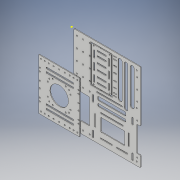
# Autodesk Inventor part: m600backplate_28Aug
Saved by Autodesk Inventor 2019 (Build 230136000, 136)
## iProperties
Created: 2019-07-14
Part Number: m600backplate_28Aug
Material: Generic
Document SubType Name: Modeling
Designer: Dell
Density: 1 g/cm^3
Appearance: Default
Author: Dell
Autodesk Inventor part; units mm, degrees
(part 1 of 2)
ref_plane "YZ Plane" through (0, 0, 0) normal (1, 0, 0) x (0, 1, 0)
ref_plane "XZ Plane" through (0, 0, 0) normal (0, 1, 0) x (-1, 0, 0)
ref_plane "XY Plane" through (0, 0, 0) normal (0, 0, 1) x (1, 0, 0)
sketch "Sketch1" plane through (0, 0, 0) normal (0, 0, 1) x (1, 0, 0)
  point P0 (0, 0)
sketch "Sketch2" plane through (0, 0, 0) normal (0, 0, 1) x (1, 0, 0)
  point P0 (0, 0)
sketch "Sketch3" plane through (0, 0, 0) normal (0, 0, 1) x (1, 0, 0)
  line L0 (0, 0) -> (190, 0)
  line L1 (190, 0) -> (190, -240)
  line L2 (190, -240) -> (0, -240)
  line L3 (0, -240) -> (0, 0)
  dimension "d0" = 190
  dimension "d1" = 240
  constraints: 8 end point, 2 parallel, 1 horizontal, 1 perpendicular
  measures "d0" distance of L1.end L2.end
  measures "d1" distance of L0.end L1.end
extrude "Extrusion1" add sketch "Sketch3" along normal blind 2
sketch "Sketch4" plane through (0, 0, 2) normal (0, 0, 1) x (1, 0, 0)
  line L0 (190, 0) -> (0, 0) projected
  line L1 (190, 0) -> (179.65, 0)
  line L2 (179.65, 0) -> (179.65, -13)
  line L3 (179.65, -13) -> (190, -13)
  line L4 (190, -13) -> (190, 0)
  line L5 (0, -240) -> (190, -240) projected
  line L6 (190, -240) -> (179.65, -240)
  line L7 (179.65, -240) -> (179.65, -230)
  line L8 (179.65, -230) -> (190, -230)
  line L9 (190, -230) -> (190, -240)
  circle A0 centre (179.65, -13) radius 1.75
  circle A1 centre (179.65, -230) radius 1.75
  line L10 (190, 0) -> (50.325, 0)
  line L11 (50.325, 0) -> (50.325, -10)
  line L12 (190, -10) -> (190, 0)
  line L13 (50.325, 0) -> (32.255, 0)
  line L14 (32.255, 0) -> (32.255, -10)
  line L15 (50.325, -10) -> (50.325, 0)
  line L16 (190, -240) -> (50.325, -240)
  line L17 (50.325, -240) -> (50.325, -230)
  line L18 (50.325, -230) -> (190, -230)
  line L19 (190, -230) -> (190, -240)
  line L20 (50.325, -240) -> (32.255, -240)
  line L21 (32.255, -240) -> (32.255, -230)
  line L22 (32.255, -230) -> (50.325, -230)
  line L23 (50.325, -230) -> (50.325, -240)
  circle A2 centre (50.325, -230) radius 1.75
  circle A3 centre (32.255, -230) radius 1.75
  line L24 (190, 0) -> (50.325, 0)
  line L25 (50.325, 0) -> (50.325, -13)
  line L26 (50.325, -13) -> (190, -13)
  line L27 (190, -13) -> (190, 0)
  line L28 (190, 0) -> (32.255, 0)
  line L29 (32.255, 0) -> (32.255, -13)
  line L30 (32.255, -13) -> (190, -13)
  line L31 (190, -13) -> (190, 0)
  circle A4 centre (32.255, -13) radius 1.75
  circle A5 centre (50.325, -13) radius 1.75
  line L32 (32.255, -13) -> (15.255, -13)
  circle A6 centre (15.255, -13) radius 1.75
  line L33 (190, -13) -> (179.65, -13)
  line L34 (179.65, -13) -> (179.65, -43)
  line L35 (179.65, -43) -> (190, -43)
  line L36 (190, -43) -> (190, -13)
  line L37 (179.65, -13) -> (50.325, -13)
  line L38 (50.325, -13) -> (50.325, -42.7133)
  line L39 (50.325, -42.7133) -> (179.65, -42.7133)
  line L40 (179.65, -42.7133) -> (179.65, -13)
  line L41 (50.325, -13) -> (32.255, -13)
  line L42 (32.255, -13) -> (32.255, -42.7133)
  line L43 (32.255, -42.7133) -> (50.325, -42.7133)
  line L44 (50.325, -42.7133) -> (50.325, -13)
  line L45 (32.255, -13) -> (15.255, -13)
  line L46 (15.255, -13) -> (15.255, -42.7133)
  line L47 (15.255, -42.7133) -> (32.255, -42.7133)
  line L48 (32.255, -42.7133) -> (32.255, -13)
  line L49 (190, -43) -> (179.65, -43)
  line L50 (179.65, -43) -> (179.65, -73)
  line L51 (179.65, -73) -> (190, -73)
  line L52 (190, -73) -> (190, -43)
  line L53 (179.65, -43) -> (50.325, -43)
  line L54 (50.325, -43) -> (50.325, -73)
  line L55 (50.325, -73) -> (179.65, -73)
  line L56 (179.65, -73) -> (179.65, -43)
  line L57 (50.325, -43) -> (32.255, -43)
  line L58 (32.255, -43) -> (32.255, -73)
  line L59 (32.255, -73) -> (50.325, -73)
  line L60 (50.325, -73) -> (50.325, -43)
  line L61 (32.255, -43) -> (15.255, -43)
  line L62 (15.255, -43) -> (15.255, -73)
  line L63 (15.255, -73) -> (32.255, -73)
  line L64 (32.255, -73) -> (32.255, -43)
  line L65 (190, -73) -> (179.65, -73)
  line L66 (179.65, -73) -> (179.65, -103)
  line L67 (179.65, -103) -> (190, -103)
  line L68 (190, -103) -> (190, -73)
  line L69 (179.65, -73) -> (50.325, -73)
  line L70 (50.325, -73) -> (50.325, -103)
  line L71 (50.325, -103) -> (179.65, -103)
  line L72 (179.65, -103) -> (179.65, -73)
  line L73 (50.325, -73) -> (32.255, -73)
  line L74 (32.255, -73) -> (32.255, -103)
  line L75 (32.255, -103) -> (50.325, -103)
  line L76 (50.325, -103) -> (50.325, -73)
  line L77 (32.255, -73) -> (15.255, -73)
  line L78 (15.255, -73) -> (15.255, -103)
  line L79 (15.255, -103) -> (32.255, -103)
  line L80 (32.255, -103) -> (32.255, -73)
  circle A7 centre (179.65, -43) radius 1.75
  circle A8 centre (179.65, -73) radius 1.75
  circle A9 centre (179.65, -103) radius 1.75
  circle A10 centre (50.325, -43) radius 1.75
  circle A11 centre (32.255, -43) radius 1.75
  circle A12 centre (15.255, -43) radius 1.75
  circle A13 centre (50.325, -73) radius 1.75
  circle A14 centre (32.255, -73) radius 1.75
  circle A15 centre (15.255, -73) radius 1.75
  circle A16 centre (15.255, -103) radius 1.75
  circle A17 centre (32.255, -103) radius 1.75
  circle A18 centre (50.325, -103) radius 1.75
  line L81 (50.325, -13) -> (53.325, -13)
  line L82 (53.325, -13) -> (53.325, -8)
  line L83 (53.325, -8) -> (50.325, -8)
  line L84 (50.325, -8) -> (50.325, -13)
  line L85 (53.325, -8) -> (112.325, -8)
  line L86 (112.325, -8) -> (112.325, -92.2031)
  line L87 (112.325, -92.2031) -> (53.325, -92.2031)
  line L88 (53.325, -92.2031) -> (53.325, -8)
  line L89 (53.325, -8) -> (112.325, -8)
  line L90 (112.325, -8) -> (112.325, -111)
  line L91 (112.325, -111) -> (53.325, -111)
  line L92 (53.325, -111) -> (53.325, -8)
  line L93 (50.325, -13) -> (127.325, -13)
  line L94 (127.325, -13) -> (127.325, -58)
  line L95 (127.325, -58) -> (50.325, -58)
  line L96 (50.325, -58) -> (50.325, -13)
  line L97 (127.325, -58) -> (112.325, -58)
  line L98 (112.325, -58) -> (112.325, -18.0003)
  line L99 (112.325, -18.0003) -> (127.325, -18.0003)
  line L100 (127.325, -18.0003) -> (127.325, -58)
  line L101 (127.325, -58) -> (112.325, -58)
  line L102 (112.325, -58) -> (112.325, -97.9958)
  line L103 (112.325, -97.9958) -> (127.325, -97.9958)
  line L104 (127.325, -97.9958) -> (127.325, -58)
  line L105 (116.2641, -18.0003) -> (123.5774, -18.0003) construction
  line L106 (116.2641, -19.0003) -> (123.5774, -19.0003)
  line L107 (123.5774, -17.0003) -> (116.2641, -17.0003)
  arc A19 (116.2641, -17.0003) -> (116.2641, -19.0003) centre (116.2641, -18.0003) ccw
  arc A20 (123.5774, -19.0003) -> (123.5774, -17.0003) centre (123.5774, -18.0003) ccw
  line L108 (116.2641, -97.9958) -> (123.5774, -97.9958) construction
  line L109 (116.2641, -98.9958) -> (123.5774, -98.9958)
  line L110 (123.5774, -96.9958) -> (116.2641, -96.9958)
  arc A21 (116.2641, -96.9958) -> (116.2641, -98.9958) centre (116.2641, -97.9958) ccw
  arc A22 (123.5774, -98.9958) -> (123.5774, -96.9958) centre (123.5774, -97.9958) ccw
  line L111 (116.2641, -10.5) -> (123.5774, -10.5) construction
  line L112 (116.2641, -11.5) -> (123.5774, -11.5)
  line L113 (123.5774, -9.5) -> (116.2641, -9.5)
  arc A23 (116.2641, -9.5) -> (116.2641, -11.5) centre (116.2641, -10.5) ccw
  arc A24 (123.5774, -11.5) -> (123.5774, -9.5) centre (123.5774, -10.5) ccw
  line L114 (116.2641, -104.75) -> (123.5774, -104.75) construction
  line L115 (116.2641, -105.75) -> (123.5774, -105.75)
  line L116 (123.5774, -103.75) -> (116.2641, -103.75)
  arc A25 (116.2641, -103.75) -> (116.2641, -105.75) centre (116.2641, -104.75) ccw
  arc A26 (123.5774, -105.75) -> (123.5774, -103.75) centre (123.5774, -104.75) ccw
  line L117 (50.325, -103) -> (32.255, -103)
  line L118 (32.255, -103) -> (32.255, -128)
  line L119 (32.255, -128) -> (50.325, -128)
  line L120 (50.325, -128) -> (50.325, -103)
  circle A27 centre (50.325, -128) radius 1.75
  circle A28 centre (32.255, -128) radius 1.75
  line L121 (190, -240) -> (190, 0) projected
  line L122 (190, -240) -> (181, -240)
  line L123 (181, -240) -> (181, -219.8278)
  line L124 (181, -219.8278) -> (190, -219.8278)
  line L125 (190, -219.8278) -> (190, -240)
  circle A29 centre (181, -219.8278) radius 1.75
  line L126 (116.9207, -32.9136) -> (122.9207, -32.9136) construction
  line L127 (116.9207, -34.2126) -> (122.9207, -34.2126)
  line L128 (122.9207, -31.6146) -> (116.9207, -31.6146)
  arc A30 (116.9207, -31.6146) -> (116.9207, -34.2126) centre (116.9207, -32.9136) ccw
  arc A31 (122.9207, -34.2126) -> (122.9207, -31.6146) centre (122.9207, -32.9136) ccw
  line L129 (116.9207, -49.8149) -> (122.9207, -49.8149) construction
  line L130 (116.9207, -51.1246) -> (122.9207, -51.1246)
  line L131 (122.9207, -48.5051) -> (116.9207, -48.5051)
  arc A32 (116.9207, -48.5051) -> (116.9207, -51.1246) centre (116.9207, -49.8149) ccw
  arc A33 (122.9207, -51.1246) -> (122.9207, -48.5051) centre (122.9207, -49.8149) ccw
  line L132 (116.9207, -68.5514) -> (122.9207, -68.5514) construction
  line L133 (116.9207, -69.571) -> (122.9207, -69.571)
  line L134 (122.9207, -67.5318) -> (116.9207, -67.5318)
  arc A34 (116.9207, -67.5318) -> (116.9207, -69.571) centre (116.9207, -68.5514) ccw
  arc A35 (122.9207, -69.571) -> (122.9207, -67.5318) centre (122.9207, -68.5514) ccw
  line L135 (116.9207, -84.977) -> (122.9207, -84.977) construction
  line L136 (116.9207, -86.0208) -> (122.9207, -86.0208)
  line L137 (122.9207, -83.9332) -> (116.9207, -83.9332)
  arc A36 (116.9207, -83.9332) -> (116.9207, -86.0208) centre (116.9207, -84.977) ccw
  arc A37 (122.9207, -86.0208) -> (122.9207, -83.9332) centre (122.9207, -84.977) ccw
  point P0 (119.9207, -18.0003)
  point P1 (119.9207, -97.9958)
  point P2 (119.9207, -10.5)
  point P3 (119.9207, -104.75)
  point P4 (119.9207, -32.9136)
  point P5 (119.9207, -49.8149)
  point P6 (119.9207, -68.5514)
  point P7 (119.9207, -84.977)
  dimension "d4" = 10.35
  dimension "d5" = 13
  dimension "d6" = 10.35
  dimension "d7" = 10
  dimension "d8" = 3.5
  dimension "d9" = 3.5
  dimension "d17" = 139.675
  dimension "d18" = 18.07
  dimension "d21" = 3.5
  dimension "d22" = 3.5
  dimension "d28" = 3.5
  dimension "d29" = 3.5
  dimension "d30" = 17
  dimension "d31" = 3.5
  dimension "d32" = 30
  dimension "d33" = 30
  dimension "d34" = 30
  dimension "d35" = 3.5
  dimension "d36" = 3.5
  dimension "d37" = 3.5
  dimension "d38" = 3.5
  dimension "d39" = 3.5
  dimension "d40" = 3.5
  dimension "d41" = 3.5
  dimension "d42" = 3.5
  dimension "d43" = 3.5
  dimension "d44" = 3.5
  dimension "d45" = 3.5
  dimension "d46" = 3.5
  dimension "d49" = 3
  dimension "d50" = 5
  dimension "d51" = 59
  dimension "d52" = 84.2031
  dimension "d54" = 77
  dimension "d55" = 45
  dimension "d56" = 2
  dimension "d57" = 2
  dimension "d58" = 2
  dimension "d59" = 2
  dimension "d89" = 103
  dimension "d105" = 3.5
  dimension "d106" = 3.5
  dimension "d107" = 25
  dimension "d111" = 3.5
  dimension "d112" = 9
  dimension "d148" = 6
  dimension "d149" = 6
  dimension "d150" = 7.1016
  dimension "d151" = 6
  dimension "d152" = 6
  constraints: 286 end point, 67 parallel, 38 centre point, 32 point on circle, 32 tangent, 29 horizontal, 29 perpendicular, 22 coincident, 14 point on line, 8 midpoint, 1 other
  measures "d4" distance of L3.end L2.end
  measures "d5" distance of L1.end L2.end
  measures "d6" distance of L7.end L8.end
  measures "d7" distance of L6.end L7.end
  measures "d8" diameter of A0
  measures "d9" diameter of A1
  measures "d17" distance of L12.start L11.end
  measures "d18" distance of L15.start L14.end
  measures "d21" diameter of A2
  measures "d22" diameter of A3
  measures "d28" diameter of A4
  measures "d29" diameter of A5
  measures "d30" distance of L32.start L32.end
  measures "d31" diameter of A6
  measures "d32" distance of L33.end L34.end
  measures "d33" distance of L49.end L50.end
  measures "d34" distance of L65.end L66.end
  measures "d35" diameter of A7
  measures "d36" diameter of A8
  measures "d37" diameter of A9
  measures "d38" diameter of A10
  measures "d39" diameter of A11
  measures "d40" diameter of A12
  measures "d41" diameter of A13
  measures "d42" diameter of A14
  measures "d43" diameter of A15
  measures "d44" diameter of A16
  measures "d45" diameter of A17
  measures "d46" diameter of A18
  measures "d49" distance of L83.end L82.end
  measures "d50" distance of L81.end L82.end
  measures "d51" distance of L86.end L87.end
  measures "d52" distance of L85.end L86.end
  measures "d54" distance of L94.end L95.end
  measures "d55" distance of L93.end L94.end
  measures "d56" diameter of A20
  measures "d57" diameter of A22
  measures "d58" diameter of A24
  measures "d59" diameter of A26
  measures "d89" distance of L89.end L90.end
  measures "d105" diameter of A27
  measures "d106" diameter of A28
  measures "d107" distance of L119.end L117.start
  measures "d111" diameter of A29
  measures "d112" distance of L123.end L124.end
  measures "d148" distance of L135.start L135.end
  measures "d149" distance of L132.start L132.end
  measures "d150" distance between parallel lines of L39 L129
  measures "d151" distance of L131.start L131.end
  measures "d152" distance of L126.start L126.end
extrude "Extrusion2" cut sketch "Sketch4" against normal blind 2 contours A0 L3 L2 | L2 L26 A0 | L34 A0 L26 | L3 A0 L34 | L85 L86 L26 L82 | A4 L30 L29 | L29 L32 A4 | A5 L26 L25 | L25 L30 A5 | L26 L86 L39 L88 | L42 A4 L32 | L30 A4 L42 | L38 A5 L30 | L26 A5 L38 | L39 L86 L53 L88 | A20 L106 A19 L99 | L99 A19 L107 A20 | A9 L71 L67 | L67 L66 A9 | A6 L46 L32 | L32 L46 A6 | A10 L53 L96 L39 | L39 L38 A10 | L53 L86 L95 L88 | L66 L71 A9 | A29 L123 L124 | L124 L123 A29 | A11 L43 L42 | L42 L47 A11 | L38 L43 A10 | L96 L57 A10 L43 | A10 L54 L53 | L95 L86 L55 L88 | L90 L91 L92 L71 | L71 L92 L87 L90 | A1 L123 L8 | L8 L123 A1 | L43 A11 L57 L61 L47 | A12 L47 L46 | L46 L47 A12 L61 L62 | L54 A10 L57 | L55 L86 L87 L88 | L123 A1 L7 L8 | L8 L18 A1 L123 | A11 L58 L57 | L61 L58 A11 | L62 L61 A12 | A13 L70 L55 | L55 L54 A13 | L54 L59 A13 | A22 L109 A21 L103 | L103 A21 L110 A22 | A18 L120 L71 | L71 L70 A18 | L7 A1 L18 | A15 L63 L62 | L62 L78 A15 | L70 A13 L59 | L75 A18 L70 | L120 A18 L75 | A2 L17 L18 | L18 L22 A2 | A14 L59 L58 | L58 L63 A14 | L63 A15 L78 | A14 L74 L59 | A27 L119 L120 | L120 L119 A27 | L17 A2 L22 | L74 A14 L63 | A16 L79 L78 | L78 L79 A16 | A17 L118 L75 | L75 L74 A17 | A3 L21 L22 | L22 L21 A3 | L74 L79 A17 | L118 A17 L79 | A28 L118 L119 | L119 L118 A28 | A23 L113 A24 L112 | A25 L116 A26 L115 | A30 L128 A31 L127 | A32 L131 A33 L130 | A34 L134 A35 L133 | A36 L137 A37 L136
sketch "Sketch5" plane through (0, 0, 2) normal (0, 0, 1) x (1, 0, 0)
  line L0 (190, 0) -> (190, -240) projected
  line L1 (190, 0) -> (181, 0)
  line L2 (181, 0) -> (181, -86.7053)
  line L3 (181, -86.7053) -> (190, -86.7053)
  line L4 (190, -86.7053) -> (190, 0)
  line L5 (190, -240) -> (181, -240)
  line L6 (181, -240) -> (181, -131.882)
  line L7 (181, -131.882) -> (190, -131.882)
  line L8 (190, -131.882) -> (190, -240)
  circle A0 centre (181, -86.7053) radius 1.75
  circle A1 centre (181, -131.882) radius 1.75
  line L9 (190, 0) -> (181, 0)
  line L10 (181, 0) -> (181, -28.9003)
  line L11 (181, -28.9003) -> (190, -28.9003)
  line L12 (190, -28.9003) -> (190, 0)
  line L13 (190, -28.9003) -> (181, -28.9003)
  line L14 (181, -28.9003) -> (181, -58.2669)
  line L15 (181, -58.2669) -> (190, -58.2669)
  line L16 (190, -58.2669) -> (190, -28.9003)
  circle A2 centre (181, -28.9003) radius 1.75
  circle A3 centre (181, -58.2669) radius 1.75
  point P0 (0, 0)
  dimension "d12" = 9
  dimension "d13" = 3.5
  dimension "d14" = 3.5
  dimension "d47" = 3.5
  dimension "d48" = 3.5
  constraints: 32 end point, 8 parallel, 4 centre point, 4 coincident, 4 horizontal, 4 perpendicular, 3 point on line
  measures "d12" distance of L3.end L2.end
  measures "d13" diameter of A0
  measures "d14" diameter of A1
  measures "d47" diameter of A2
  measures "d48" diameter of A3
extrude "Extrusion3" cut sketch "Sketch5" against normal blind 2 contours A2 L2 L11 | L11 L2 A2 | L2 A2 | A3 L2 L15 | L15 L2 A3 | A0 L2 L3 | L3 L2 A0 | L2 A3 | A1 L6 L7 | L7 L6 A1
sketch "Sketch6" plane through (0, 0, 2) normal (0, 0, 1) x (1, 0, 0)
  line L0 (0, 0) -> (25, 0)
  line L1 (25, 0) -> (25, -108)
  line L2 (25, -108) -> (0, -108)
  line L3 (0, -108) -> (0, 0)
  circle A0 centre (32.255, -10) radius 1.75 projected
  line L4 (0, -108) -> (25, -108)
  line L5 (25, -108) -> (25, -240)
  line L6 (25, -240) -> (0, -240)
  line L7 (0, -240) -> (0, -108)
  line L8 (190, 0) -> (0, 0) projected
  line L9 (0, 0) -> (7.255, 0)
  line L10 (7.255, 0) -> (7.255, -108)
  line L11 (7.255, -108) -> (0, -108)
  line L12 (0, -108) -> (0, 0)
  line L13 (0, 0) -> (0, -240) projected
  line L14 (0, 0) -> (50.325, 0)
  line L15 (50.325, 0) -> (50.325, -160)
  line L16 (50.325, -160) -> (0, -160)
  line L17 (0, -160) -> (0, 0)
  line L18 (0, -160) -> (50.325, -160)
  line L19 (50.325, -160) -> (50.325, -210)
  line L20 (50.325, -210) -> (0, -210)
  line L21 (0, -210) -> (0, -160)
  line L22 (190, -159.8282) -> (179.65, -159.8282)
  line L23 (179.65, -159.8282) -> (179.65, -210.3723)
  line L24 (179.65, -210.3723) -> (190, -210.3723)
  line L25 (190, -210.3723) -> (190, -159.8282)
  dimension "d23" = 108
  dimension "d24" = 25
  dimension "d53" = 7.255
  dimension "d60" = 160
  dimension "d61" = 50
  constraints: 48 end point, 12 parallel, 6 horizontal, 6 perpendicular, 1 point on line
  measures "d23" distance of L0.end L1.end
  measures "d24" distance of L1.end L2.end
  measures "d53" distance of L10.end L11.end
  measures "d60" distance of L14.end L15.end
  measures "d61" distance of L18.end L19.end
extrude "Extrusion4" cut sketch "Sketch6" against normal blind 10 contours L0 L10 L2 L3 | L2 L5 L16 L7 | L16 L5 L20 L7 | L20 L5 L6 L7 | L16 L19 L20 L5 | L25 L24 L23 L22
sketch "Sketch7" plane through (38.9808, -119.1264, 2) normal (0, 0, 1) x (1, 0, 0)
  line L0 (150, -215) -> (150, 0)
  line L1 (150, 0) -> (129.155, 0)
  line L2 (129.155, 0) -> (129.155, -12.875)
  line L3 (129.155, -12.875) -> (150, -12.875)
  line L4 (150, -12.875) -> (150, 0)
  line L5 (0, 0) -> (20.845, 0)
  line L6 (20.845, 0) -> (20.845, -12.875)
  line L7 (20.845, -12.875) -> (0, -12.875)
  line L8 (0, -12.875) -> (0, 0)
  circle A0 centre (129.155, -12.875) radius 1.75
  circle A1 centre (20.845, -12.875) radius 1.75
  line L9 (150, 0) -> (129.155, 0)
  line L10 (129.155, 0) -> (129.155, -97.755)
  line L11 (129.155, -97.755) -> (150, -97.755)
  line L12 (150, -97.755) -> (150, 0)
  line L13 (0, 0) -> (20.845, 0)
  line L14 (20.845, 0) -> (20.845, -97.755)
  line L15 (20.845, -97.755) -> (0, -97.755)
  line L16 (0, -97.755) -> (0, 0)
  circle A2 centre (20.845, -97.755) radius 1.75
  circle A3 centre (129.155, -97.755) radius 1.75
  line L17 (150, 0) -> (0, 0)
  line L18 (0, 0) -> (20.845, 0)
  line L19 (20.845, 0) -> (20.845, -27.95)
  line L20 (20.845, -27.95) -> (0, -27.95)
  line L21 (0, -27.95) -> (0, 0)
  circle A4 centre (20.845, -27.95) radius 1.75
  line L22 (150, 0) -> (129.155, 0)
  line L23 (129.155, 0) -> (129.155, -27.95)
  line L24 (129.155, -27.95) -> (150, -27.95)
  line L25 (150, -27.95) -> (150, 0)
  circle A5 centre (129.155, -27.95) radius 1.75
  line L26 (0, -97.755) -> (20.845, -97.755)
  line L27 (20.845, -97.755) -> (20.845, -112.83)
  line L28 (20.845, -112.83) -> (0, -112.83)
  line L29 (0, -112.83) -> (0, -97.755)
  line L30 (150, -97.755) -> (129.155, -97.755)
  line L31 (129.155, -97.755) -> (129.155, -112.83)
  line L32 (129.155, -112.83) -> (150, -112.83)
  line L33 (150, -112.83) -> (150, -97.755)
  circle A6 centre (20.845, -112.83) radius 1.75
  circle A7 centre (129.155, -112.83) radius 1.75
  line L34 (20.845, -12.875) -> (20.845, -27.95) construction
  line L35 (19.095, -12.875) -> (19.095, -27.95)
  line L36 (22.595, -27.95) -> (22.595, -12.875)
  arc A8 (22.595, -12.875) -> (19.095, -12.875) centre (20.845, -12.875) ccw
  arc A9 (19.095, -27.95) -> (22.595, -27.95) centre (20.845, -27.95) ccw
  line L37 (129.155, -27.95) -> (129.1553, -12.8747) construction
  line L38 (130.905, -27.95) -> (130.9053, -12.8747)
  line L39 (127.4053, -12.8746) -> (127.405, -27.95)
  arc A10 (127.405, -27.95) -> (130.905, -27.95) centre (129.155, -27.95) ccw
  arc A11 (130.9053, -12.8747) -> (127.4053, -12.8746) centre (129.1553, -12.8747) ccw
  line L40 (129.155, -97.755) -> (129.155, -112.83) construction
  line L41 (127.405, -97.755) -> (127.405, -112.83)
  line L42 (130.905, -112.83) -> (130.905, -97.755)
  arc A12 (130.905, -97.755) -> (127.405, -97.755) centre (129.155, -97.755) ccw
  arc A13 (127.405, -112.83) -> (130.905, -112.83) centre (129.155, -112.83) ccw
  line L43 (20.845, -97.755) -> (20.845, -112.83) construction
  line L44 (19.095, -97.755) -> (19.095, -112.83)
  line L45 (22.595, -112.83) -> (22.595, -97.755)
  arc A14 (22.595, -97.755) -> (19.095, -97.755) centre (20.845, -97.755) ccw
  arc A15 (19.095, -112.83) -> (22.595, -112.83) centre (20.845, -112.83) ccw
  line L46 (42.3212, -18.1679) -> (102.3212, -18.1679) construction
  line L47 (42.3212, -19.6679) -> (102.3212, -19.6679)
  line L48 (102.3212, -16.6679) -> (42.3212, -16.6679)
  arc A16 (42.3212, -16.6679) -> (42.3212, -19.6679) centre (42.3212, -18.1679) ccw
  arc A17 (102.3212, -19.6679) -> (102.3212, -16.6679) centre (102.3212, -18.1679) ccw
  arc A18 (118.7811, -14.3736) -> (118.7811, -11.3736) centre (118.7811, -12.8736) ccw
  line L49 (31.9307, 0) -> (99.9307, 0) construction
  line L50 (31.9307, -1.5) -> (99.9307, -1.5)
  line L51 (99.9307, 1.5) -> (31.9307, 1.5)
  arc A19 (31.9307, 1.5) -> (31.9307, -1.5) centre (31.9307, 0) ccw
  arc A20 (99.9307, -1.5) -> (99.9307, 1.5) centre (99.9307, 0) ccw
  line L52 (42.3212, -44.7177) -> (102.3212, -44.7177) construction
  line L53 (42.3212, -46.2177) -> (102.3212, -46.2177)
  line L54 (102.3212, -43.2177) -> (42.3212, -43.2177)
  arc A21 (42.3212, -43.2177) -> (42.3212, -46.2177) centre (42.3212, -44.7177) ccw
  arc A22 (102.3212, -46.2177) -> (102.3212, -43.2177) centre (102.3212, -44.7177) ccw
  line L55 (90.1611, 94.0299) -> (90.1611, 77.0497) construction
  line L56 (87.6611, 94.0299) -> (87.6611, 77.0497)
  line L57 (92.6611, 77.0497) -> (92.6611, 94.0299)
  arc A23 (92.6611, 94.0299) -> (87.6611, 94.0299) centre (90.1611, 94.0299) ccw
  arc A24 (87.6611, 77.0497) -> (92.6611, 77.0497) centre (90.1611, 77.0497) ccw
  line L58 (90.1611, 48.3141) -> (90.1611, 31.2392) construction
  line L59 (88.8111, 48.3141) -> (88.8111, 31.2392)
  line L60 (91.5111, 31.2392) -> (91.5111, 48.3141)
  arc A25 (91.5111, 48.3141) -> (88.8111, 48.3141) centre (90.1611, 48.3141) ccw
  arc A26 (88.8111, 31.2392) -> (91.5111, 31.2392) centre (90.1611, 31.2392) ccw
  line L61 (131.941, 94.0299) -> (131.941, 77.0497) construction
  line L62 (130.591, 94.0299) -> (130.591, 77.0497)
  line L63 (133.291, 77.0497) -> (133.291, 94.0299)
  arc A27 (133.291, 94.0299) -> (130.591, 94.0299) centre (131.941, 94.0299) ccw
  arc A28 (130.591, 77.0497) -> (133.291, 77.0497) centre (131.941, 77.0497) ccw
  line L64 (131.941, 48.3141) -> (131.941, 31.2392) construction
  line L65 (130.591, 48.3141) -> (130.591, 31.2392)
  line L66 (133.291, 31.2392) -> (133.291, 48.3141)
  arc A29 (133.291, 48.3141) -> (130.591, 48.3141) centre (131.941, 48.3141) ccw
  arc A30 (130.591, 31.2392) -> (133.291, 31.2392) centre (131.941, 31.2392) ccw
  line L67 (112.7117, 142.4796) -> (112.7117, 43.0119) construction
  line L68 (26.4237, -54.8428) -> (26.4237, -84.9666) construction
  line L69 (25.0737, -54.8428) -> (25.0737, -84.9666)
  line L70 (27.7737, -84.9666) -> (27.7737, -54.8428)
  arc A31 (27.7737, -54.8428) -> (25.0737, -54.8428) centre (26.4237, -54.8428) ccw
  arc A32 (25.0737, -84.9666) -> (27.7737, -84.9666) centre (26.4237, -84.9666) ccw
  line L71 (51.0407, -54.8428) -> (51.0407, -84.9666) construction
  line L72 (49.6907, -54.8428) -> (49.6907, -84.9666)
  line L73 (52.3907, -84.9666) -> (52.3907, -54.8428)
  arc A33 (52.3907, -54.8428) -> (49.6907, -54.8428) centre (51.0407, -54.8428) ccw
  arc A34 (49.6907, -84.9666) -> (52.3907, -84.9666) centre (51.0407, -84.9666) ccw
  line L74 (73.6712, -54.8428) -> (73.6712, -84.9666) construction
  line L75 (72.3212, -54.8428) -> (72.3212, -84.9666)
  line L76 (75.0212, -84.9666) -> (75.0212, -54.8428)
  arc A35 (75.0212, -54.8428) -> (72.3212, -54.8428) centre (73.6712, -54.8428) ccw
  arc A36 (72.3212, -84.9666) -> (75.0212, -84.9666) centre (73.6712, -84.9666) ccw
  line L77 (51.0407, -54.8428) -> (51.0407, -84.9666) construction
  line L78 (49.6907, -54.8428) -> (49.6907, -84.9666)
  line L79 (52.3907, -84.9666) -> (52.3907, -54.8428)
  arc A37 (52.3907, -54.8428) -> (49.6907, -54.8428) centre (51.0407, -54.8428) ccw
  arc A38 (49.6907, -84.9666) -> (52.3907, -84.9666) centre (51.0407, -84.9666) ccw
  line L80 (95.5512, -54.8428) -> (95.5512, -84.9666) construction
  line L81 (94.2012, -54.8428) -> (94.2012, -84.9666)
  line L82 (96.9012, -84.9666) -> (96.9012, -54.8428)
  arc A39 (96.9012, -54.8428) -> (94.2012, -54.8428) centre (95.5512, -54.8428) ccw
  arc A40 (94.2012, -84.9666) -> (96.9012, -84.9666) centre (95.5512, -84.9666) ccw
  line L83 (118.7811, -54.8428) -> (118.7811, -84.9666) construction
  line L84 (117.4311, -54.8428) -> (117.4311, -84.9666)
  line L85 (120.1311, -84.9666) -> (120.1311, -54.8428)
  arc A41 (120.1311, -54.8428) -> (117.4311, -54.8428) centre (118.7811, -54.8428) ccw
  arc A42 (117.4311, -84.9666) -> (120.1311, -84.9666) centre (118.7811, -84.9666) ccw
  line L86 (41.7212, -105.2925) -> (72.3212, -105.2925) construction
  line L87 (41.7212, -106.6425) -> (72.3212, -106.6425)
  line L88 (72.3212, -103.9425) -> (41.7212, -103.9425)
  arc A43 (41.7212, -103.9425) -> (41.7212, -106.6425) centre (41.7212, -105.2925) ccw
  arc A44 (72.3212, -106.6425) -> (72.3212, -103.9425) centre (72.3212, -105.2925) ccw
  line L89 (85.8075, -105.2925) -> (114.0617, -105.2925) construction
  line L90 (85.8075, -106.6425) -> (114.0617, -106.6425)
  line L91 (114.0617, -103.9425) -> (85.8075, -103.9425)
  arc A45 (85.8075, -103.9425) -> (85.8075, -106.6425) centre (85.8075, -105.2925) ccw
  arc A46 (114.0617, -106.6425) -> (114.0617, -103.9425) centre (114.0617, -105.2925) ccw
  line L92 (34.0582, -32.545) -> (110.4432, -32.545)
  line L93 (110.4432, -32.545) -> (110.4432, -25.545)
  line L94 (110.4432, -25.545) -> (34.0582, -25.545)
  line L95 (34.0582, -25.545) -> (34.0582, -32.545)
  line L96 (41.7212, -54.8428) -> (107.4704, -54.8428)
  line L97 (107.4704, -54.8428) -> (107.4704, -89.7612)
  line L98 (107.4704, -89.7612) -> (41.7212, -89.7612)
  line L99 (41.7212, -89.7612) -> (41.7212, -54.8428)
  line L100 (34.0582, -8.1679) -> (110.4432, -8.1679)
  line L101 (110.4432, -8.1679) -> (110.4432, -18.1679)
  line L102 (110.4432, -18.1679) -> (34.0582, -18.1679)
  line L103 (34.0582, -18.1679) -> (34.0582, -8.1679)
  point P0 (20.845, -20.4125)
  point P1 (129.1551, -20.4123)
  point P2 (129.155, -105.2925)
  point P3 (20.845, -105.2925)
  point P4 (72.3212, -18.1679)
  point P5 (78.3906, -12.8736)
  point P6 (73.5055, -43.6458)
  point P7 (78.3897, -58.1242)
  point P8 (78.3906, -80.4309)
  point P9 (65.9307, 0)
  point P10 (72.3212, -44.7177)
  point P11 (90.1611, 85.5398)
  point P12 (90.1611, 39.7766)
  point P13 (131.941, 85.5398)
  point P14 (131.941, 39.7766)
  point P15 (112.7117, 92.7458)
  point P16 (26.4237, -69.9047)
  point P17 (51.0407, -69.9047)
  point P18 (73.6712, -69.9047)
  point P19 (51.0407, -69.9047)
  point P20 (95.5512, -69.9047)
  point P21 (118.7811, -69.9047)
  point P22 (57.0212, -105.2925)
  point P23 (99.9346, -105.2925)
  dimension "d79" = 20.845
  dimension "d80" = 12.875
  dimension "d77" = 20.845
  dimension "d78" = 12.875
  dimension "d76" = 3.5
  dimension "d75" = 3.5
  dimension "d74" = 97.755
  dimension "d72" = 3.5
  dimension "d71" = 3.5
  dimension "d70" = 27.95
  dimension "d69" = 3.5
  dimension "d68" = 27.95
  dimension "d67" = 20.845
  dimension "d66" = 3.5
  dimension "d73" = 97.755
  dimension "d65" = 15.075
  dimension "d64" = 3.5
  dimension "d63" = 3.5
  dimension "d62" = 3.5
  dimension "d84" = 3
  dimension "d85" = 3
  dimension "d90" = 3
  dimension "d91" = 3
  dimension "d92" = 5
  dimension "d93" = 2.7
  dimension "d94" = 2.7
  dimension "d95" = 2.7
  dimension "d97" = 2.7
  dimension "d98" = 2.7
  dimension "d99" = 2.7
  dimension "d100" = 2.7
  dimension "d101" = 2.7
  dimension "d102" = 2.7
  dimension "d103" = 2.7
  dimension "d104" = 2.7
  dimension "d108" = 60
  dimension "d109" = 60
  dimension "d110" = 68
  dimension "d155" = 7
  dimension "d156" = 10
  constraints: 248 end point, 78 point on circle, 76 tangent, 48 parallel, 47 centre point, 20 midpoint, 14 horizontal, 12 perpendicular, 10 point on line, 9 coincident, 2 collinear, 2 concentric, 2 vertical
  measures "d79" distance of L3.end L2.end
  measures "d80" distance of L1.end L2.end
  measures "d77" distance of L6.end L7.end
  measures "d78" distance of L5.end L6.end
  measures "d76" diameter of A0
  measures "d75" diameter of A1
  measures "d74" distance of L9.end L10.end
  measures "d72" diameter of A2
  measures "d71" diameter of A3
  measures "d70" distance of L18.end L19.end
  measures "d69" diameter of A4
  measures "d68" distance of L22.end L23.end
  measures "d67" distance of L23.end L24.end
  measures "d66" diameter of A5
  measures "d73" distance of L13.end L14.end
  measures "d65" distance of L26.end L27.end
  measures "d64" diameter of A6
  measures "d63" diameter of A7
  measures "d62" diameter of A11
  measures "d84" diameter of A17
  measures "d85" diameter of A18
  measures "d90" diameter of A20
  measures "d91" diameter of A22
  measures "d92" diameter of A24
  measures "d93" diameter of A26
  measures "d94" diameter of A28
  measures "d95" diameter of A30
  measures "d97" diameter of A32
  measures "d98" diameter of A34
  measures "d99" diameter of A36
  measures "d100" diameter of A38
  measures "d101" diameter of A40
  measures "d102" diameter of A42
  measures "d103" diameter of A44
  measures "d104" diameter of A46
  measures "d108" distance of L48.start L48.end
  measures "d109" distance of L54.start L54.end
  measures "d110" distance of L51.start L51.end
  measures "d155" distance of L94.end L92.start
  measures "d156" distance of L100.end L101.end
extrude "Extrusion5" cut sketch "Sketch7" against normal blind 2 contours A20 L50 A19 L17 | L17 A19 L51 A20 | A7 L31 L32 | L32 L31 A7 | A7 L31 A3 L42 | A3 L31 L11 | L11 L10 A3 | L41 A3 L31 A7 | A5 L10 L24 | L24 L10 A5 | A5 L10 A0 L38 | L31 A3 L10 | A0 L10 L3 | L3 L2 A0 | L10 A5 | A5 L39 A0 L10 | L10 A0 L2 | A1 L14 L6 | L6 L7 A1 | L14 A1 L7 | L36 A4 L14 A1 | A1 L14 A4 L35 | A4 L14 | A4 L14 L20 | L20 L14 A4 | A2 L14 L15 | L15 L27 A2 | A2 L27 A6 L44 | A2 L27 L14 | A2 L45 A6 L27 | A6 L27 L28 | L28 L27 A6 | L102 L103 L100 L101 A17 L48 A16 | A16 L48 A17 L102 | A21 L54 A22 L53 | A31 L70 A32 L69 | L96 L73 A34 L72 | L72 A34 L73 L96 L75 A36 L76 L81 A40 L82 L97 L98 L99 | L96 L76 A36 L75 | L96 L82 A40 L81 | A41 L85 A42 L84 | A43 L88 A44 L87 | A45 L91 A46 L90 | L95 L94 L93 L92
sketch "Sketch8" plane through (0, 0, 2) normal (0, 0, 1) x (1, 0, 0)
  line L0 (56.6375, -10.4648) -> (109.4375, -10.4648)
  line L1 (109.4375, -10.4648) -> (109.4375, -108.4648)
  line L2 (109.4375, -108.4648) -> (56.6375, -108.4648)
  line L3 (56.6375, -108.4648) -> (56.6375, -10.4648)
  line L4 (112.325, -8) -> (53.325, -8) projected
  line L5 (79.8909, -10.4648) -> (80.8125, -10.4648)
  line L6 (80.8125, -10.4648) -> (80.8125, -8)
  line L7 (80.8125, -8) -> (79.8909, -8)
  line L8 (79.8909, -8) -> (79.8909, -10.4648)
  point P0 (0, 0)
  dimension "d115" = 98
  dimension "d116" = 52.8
  constraints: 16 end point, 4 parallel, 2 horizontal, 2 perpendicular, 2 point on line
  measures "d115" distance of L2.end L0.start
  measures "d116" distance of L0.start L0.end
extrude "Extrusion6" add sketch "Sketch8" against normal blind 2
sketch "Sketch9" plane through (0, 0, 2) normal (0, 0, 1) x (1, 0, 0)
  line L0 (56.6375, -108.4648) -> (56.6375, -10.4648) projected
  line L1 (56.6375, -10.4648) -> (61.1375, -10.4648)
  line L2 (61.1375, -10.4648) -> (61.1375, -13.5698)
  line L3 (61.1375, -13.5698) -> (56.6375, -13.5698)
  line L4 (56.6375, -13.5698) -> (56.6375, -10.4648)
  line L5 (56.6375, -10.4648) -> (109.4375, -10.4648) projected
  line L6 (109.4375, -10.4648) -> (104.9375, -10.4648)
  line L7 (104.9375, -10.4648) -> (104.9375, -13.5698)
  line L8 (104.9375, -13.5698) -> (109.4375, -13.5698)
  line L9 (109.4375, -13.5698) -> (109.4375, -10.4648)
  line L10 (109.4375, -108.4648) -> (56.6375, -108.4648) projected
  line L11 (109.4375, -108.4648) -> (104.9375, -108.4648)
  line L12 (104.9375, -108.4648) -> (104.9375, -105.3598)
  line L13 (104.9375, -105.3598) -> (109.4375, -105.3598)
  line L14 (109.4375, -105.3598) -> (109.4375, -108.4648)
  line L15 (56.6375, -108.4648) -> (61.1375, -108.4648)
  line L16 (61.1375, -108.4648) -> (61.1375, -105.3598)
  line L17 (61.1375, -105.3598) -> (56.6375, -105.3598)
  line L18 (56.6375, -105.3598) -> (56.6375, -108.4648)
  circle A0 centre (104.9375, -13.5698) radius 1.6
  circle A1 centre (61.1375, -13.5698) radius 1.6
  circle A2 centre (104.9375, -105.3598) radius 1.6
  circle A3 centre (61.1375, -105.3598) radius 1.6
  line L19 (103.3375, -24.1824) -> (103.3375, -40.848) construction
  line L20 (101.7375, -24.1824) -> (101.7375, -40.848)
  line L21 (104.9375, -40.848) -> (104.9375, -24.1824)
  arc A4 (104.9375, -24.1824) -> (101.7375, -24.1824) centre (103.3375, -24.1824) ccw
  arc A5 (101.7375, -40.848) -> (104.9375, -40.848) centre (103.3375, -40.848) ccw
  line L22 (103.3375, -54.0485) -> (103.3375, -71.0442) construction
  line L23 (101.7375, -54.0485) -> (101.7375, -71.0442)
  line L24 (104.9375, -71.0442) -> (104.9375, -54.0485)
  arc A6 (104.9375, -54.0485) -> (101.7375, -54.0485) centre (103.3375, -54.0485) ccw
  arc A7 (101.7375, -71.0442) -> (104.9375, -71.0442) centre (103.3375, -71.0442) ccw
  line L25 (103.3375, -83.0896) -> (103.3375, -98.6002) construction
  line L26 (101.7375, -83.0896) -> (101.7375, -98.6002)
  line L27 (104.9375, -98.6002) -> (104.9375, -83.0896)
  arc A8 (104.9375, -83.0896) -> (101.7375, -83.0896) centre (103.3375, -83.0896) ccw
  arc A9 (101.7375, -98.6002) -> (104.9375, -98.6002) centre (103.3375, -98.6002) ccw
  line L28 (62.7375, -24.1824) -> (62.7375, -40.848) construction
  line L29 (61.1375, -24.1824) -> (61.1375, -40.848)
  line L30 (64.3375, -40.848) -> (64.3375, -24.1824)
  arc A10 (64.3375, -24.1824) -> (61.1375, -24.1824) centre (62.7375, -24.1824) ccw
  arc A11 (61.1375, -40.848) -> (64.3375, -40.848) centre (62.7375, -40.848) ccw
  line L31 (62.7375, -54.0485) -> (62.7375, -71.0442) construction
  line L32 (61.1375, -54.0485) -> (61.1375, -71.0442)
  line L33 (64.3375, -71.0442) -> (64.3375, -54.0485)
  arc A12 (64.3375, -54.0485) -> (61.1375, -54.0485) centre (62.7375, -54.0485) ccw
  arc A13 (61.1375, -71.0442) -> (64.3375, -71.0442) centre (62.7375, -71.0442) ccw
  line L34 (62.7375, -83.0896) -> (62.7375, -98.6002) construction
  line L35 (61.1375, -83.0896) -> (61.1375, -98.6002)
  line L36 (64.3375, -98.6002) -> (64.3375, -83.0896)
  arc A14 (64.3375, -83.0896) -> (61.1375, -83.0896) centre (62.7375, -83.0896) ccw
  arc A15 (61.1375, -98.6002) -> (64.3375, -98.6002) centre (62.7375, -98.6002) ccw
  line L37 (72.1963, -20.8666) -> (94.5537, -20.8666) construction
  line L38 (72.1963, -22.4666) -> (94.5537, -22.4666)
  line L39 (94.5537, -19.2666) -> (72.1963, -19.2666)
  arc A16 (72.1963, -19.2666) -> (72.1963, -22.4666) centre (72.1963, -20.8666) ccw
  arc A17 (94.5537, -22.4666) -> (94.5537, -19.2666) centre (94.5537, -20.8666) ccw
  line L40 (72.1963, -33.5539) -> (94.5537, -33.5539) construction
  line L41 (72.1963, -35.1539) -> (94.5537, -35.1539)
  line L42 (94.5537, -31.9539) -> (72.1963, -31.9539)
  arc A18 (72.1963, -31.9539) -> (72.1963, -35.1539) centre (72.1963, -33.5539) ccw
  arc A19 (94.5537, -35.1539) -> (94.5537, -31.9539) centre (94.5537, -33.5539) ccw
  line L43 (72.1963, -49.9109) -> (94.5537, -49.9109) construction
  line L44 (72.1963, -51.5109) -> (94.5537, -51.5109)
  line L45 (94.5537, -48.3109) -> (72.1963, -48.3109)
  arc A20 (72.1963, -48.3109) -> (72.1963, -51.5109) centre (72.1963, -49.9109) ccw
  arc A21 (94.5537, -51.5109) -> (94.5537, -48.3109) centre (94.5537, -49.9109) ccw
  line L46 (72.1963, -66.5157) -> (94.5537, -66.5157) construction
  line L47 (72.1963, -68.1157) -> (94.5537, -68.1157)
  line L48 (94.5537, -64.9157) -> (72.1963, -64.9157)
  arc A22 (72.1963, -64.9157) -> (72.1963, -68.1157) centre (72.1963, -66.5157) ccw
  arc A23 (94.5537, -68.1157) -> (94.5537, -64.9157) centre (94.5537, -66.5157) ccw
  line L49 (72.1963, -83.0896) -> (94.5537, -83.0896) construction
  line L50 (72.1963, -84.6896) -> (94.5537, -84.6896)
  line L51 (94.5537, -81.4896) -> (72.1963, -81.4896)
  arc A24 (72.1963, -81.4896) -> (72.1963, -84.6896) centre (72.1963, -83.0896) ccw
  arc A25 (94.5537, -84.6896) -> (94.5537, -81.4896) centre (94.5537, -83.0896) ccw
  line L52 (72.1963, -97.0094) -> (94.5537, -97.0094) construction
  line L53 (72.1963, -98.6094) -> (94.5537, -98.6094)
  line L54 (94.5537, -95.4094) -> (72.1963, -95.4094)
  arc A26 (72.1963, -95.4094) -> (72.1963, -98.6094) centre (72.1963, -97.0094) ccw
  arc A27 (94.5537, -98.6094) -> (94.5537, -95.4094) centre (94.5537, -97.0094) ccw
  line L55 (53.325, -8) -> (112.325, -8) projected
  line L56 (105.6332, -10.4648) -> (106.4409, -10.4648)
  line L57 (106.4409, -10.4648) -> (106.4409, -8)
  line L58 (106.4409, -8) -> (105.6332, -8)
  line L59 (105.6332, -8) -> (105.6332, -10.4648)
  point P0 (0, 0)
  point P1 (103.3375, -32.5152)
  point P2 (103.3375, -62.5463)
  point P3 (103.3375, -90.8449)
  point P4 (62.7375, -32.5152)
  point P5 (62.7375, -62.5463)
  point P6 (62.7375, -90.8449)
  point P7 (83.375, -20.8666)
  point P8 (83.375, -33.5539)
  point P9 (83.375, -49.9109)
  point P10 (83.375, -66.5157)
  point P11 (83.375, -83.0896)
  point P12 (83.375, -97.0094)
  dimension "d117" = 4.5
  dimension "d118" = 3.105
  dimension "d119" = 4.5
  dimension "d120" = 3.105
  dimension "d121" = 4.5
  dimension "d122" = 3.105
  dimension "d123" = 3.2
  dimension "d124" = 3.2
  dimension "d125" = 3.2
  dimension "d126" = 3.2
  dimension "d129" = 3.2
  dimension "d130" = 3.2
  dimension "d131" = 3.2
  dimension "d132" = 3.2
  dimension "d133" = 3.2
  dimension "d134" = 3.2
  dimension "d135" = 3.2
  dimension "d136" = 3.2
  dimension "d137" = 3.2
  dimension "d138" = 3.2
  dimension "d139" = 3.2
  dimension "d140" = 3.2
  dimension "d143" = 3.105
  constraints: 136 end point, 48 point on circle, 48 tangent, 28 centre point, 27 parallel, 12 midpoint, 10 point on line, 7 horizontal, 5 perpendicular, 4 coincident, 1 vertical
  measures "d117" distance of L2.end L3.end
  measures "d118" distance of L1.end L2.end
  measures "d119" distance of L8.end L7.end
  measures "d120" distance of L6.end L7.end
  measures "d121" distance of L12.end L13.end
  measures "d122" distance of L11.end L12.end
  measures "d123" diameter of A0
  measures "d124" diameter of A1
  measures "d125" diameter of A2
  measures "d126" diameter of A3
  measures "d129" diameter of A5
  measures "d130" diameter of A7
  measures "d131" diameter of A9
  measures "d132" diameter of A11
  measures "d133" diameter of A13
  measures "d134" diameter of A15
  measures "d135" diameter of A17
  measures "d136" diameter of A19
  measures "d137" diameter of A21
  measures "d138" diameter of A23
  measures "d139" diameter of A25
  measures "d140" diameter of A27
  measures "d143" distance of L15.end L16.end
extrude "Extrusion7" cut sketch "Sketch9" against normal blind 2 contours A3 L16 L17 | L17 L16 A3 | A1 L2 L3 | L3 L2 A1 | A2 L13 L12 | L12 L13 A2 | A0 L8 L7 | L7 L8 A0 | A4 L21 A5 L20 | A6 L24 A7 L23 | A8 L27 A9 L26 | A10 L30 A11 L29 | A12 L33 A13 L32 | A14 L36 A15 L35 | A16 L39 A17 L38 | A18 L42 A19 L41 | A20 L45 A21 L44 | A22 L48 A23 L47 | A24 L51 A25 L50 | A26 L54 A27 L53
fillet "Fillet1" radius 2 16 edges at (109.4375, -108.4648, 1) (109.4375, -10.4648, 1) (56.6375, -10.4648, 1) (56.6375, -108.4648, 1) (190, 0, 1) (7.255, 0, 1) (25, -160, 1) (50.325, -160, 1) (50.325, -210, 1) (25, -210, 1) (25, -240, 1) (190, -240, 1) (190, -159.8282, 1) (190, -210.3723, 1) (179.65, -159.8282, 1) (179.65, -210.3723, 1)
fillet "Fillet2" radius 2 2 edges at (7.255, -108, 1) (25, -108, 1)
sketch "Sketch10" plane through (0, 0, 2) normal (0, 0, 1) x (1, 0, 0)
  line L0 (150.4718, -13.0381) -> (150.4718, -118.0381) construction
  line L1 (145.4718, -13.0381) -> (145.4718, -118.0381)
  line L2 (155.4718, -118.0381) -> (155.4718, -13.0381)
  arc A0 (155.4718, -13.0381) -> (145.4718, -13.0381) centre (150.4718, -13.0381) ccw
  arc A1 (145.4718, -118.0381) -> (155.4718, -118.0381) centre (150.4718, -118.0381) ccw
  line L3 (134.0478, -13.0381) -> (134.0478, -104.6086) construction
  line L4 (128.5408, -13.0381) -> (128.5408, -104.6086)
  line L5 (139.5548, -104.6086) -> (139.5548, -13.0381)
  arc A2 (139.5548, -13.0381) -> (128.5408, -13.0381) centre (134.0478, -13.0381) ccw
  arc A3 (128.5408, -104.6086) -> (139.5548, -104.6086) centre (134.0478, -104.6086) ccw
  line L6 (167.5133, -13.0381) -> (167.5133, -104.6086) construction
  line L7 (161.99, -13.0381) -> (161.99, -104.6086)
  line L8 (173.0365, -104.6086) -> (173.0365, -13.0381)
  arc A4 (173.0365, -13.0381) -> (161.99, -13.0381) centre (167.5133, -13.0381) ccw
  arc A5 (161.99, -104.6086) -> (173.0365, -104.6086) centre (167.5133, -104.6086) ccw
  point P0 (0, 0)
  point P1 (150.4718, -65.5381)
  point P2 (134.0478, -58.8233)
  point P3 (167.5133, -58.8233)
  dimension "d144" = 105
  dimension "d145" = 5
  constraints: 24 end point, 12 point on circle, 12 tangent, 6 centre point, 4 parallel, 3 midpoint, 2 vertical
  measures "d144" distance of L0.start L0.end
  measures "d145" radius of A0
extrude "Extrusion8" cut sketch "Sketch10" against normal blind 10
fillet "Fillet3" radius 2 8 edges at (149.4241, -144.6713, 1) (149.4241, -151.6713, 1) (73.039, -144.6713, 1) (73.039, -151.6713, 1) (73.039, -127.2943, 1) (73.039, -137.2943, 1) (149.4241, -127.2943, 1) (149.4241, -137.2943, 1)
fillet "Fillet4" radius 2 4 edges at (80.702, -173.9692, 1) (146.4512, -173.9692, 1) (80.702, -208.8876, 1) (146.4512, -208.8876, 1)
sketch "Sketch11" plane through (0, 0, 2) normal (0, 0, 1) x (1, 0, 0)
  line L0 (50.325, -208) -> (50.325, -162) projected
  line L1 (25, -158) -> (25, -110) projected
  line L2 (50.325, -162) -> (25, -162)
  line L3 (25, -162) -> (25, -140.8544)
  line L4 (25, -140.8544) -> (50.325, -140.8544)
  line L5 (50.325, -140.8544) -> (50.325, -162)
  line L6 (179.65, -161.8282) -> (179.65, -208.3723) projected
  line L7 (179.65, -161.8282) -> (191.0405, -161.8282)
  line L8 (191.0405, -161.8282) -> (191.0405, -140.8544)
  line L9 (191.0405, -140.8544) -> (179.65, -140.8544)
  line L10 (179.65, -140.8544) -> (179.65, -161.8282)
  point P0 (0, 0)
  constraints: 16 end point, 4 parallel, 2 horizontal, 2 perpendicular, 2 point on line
extrude "Extrusion9" cut sketch "Sketch11" against normal blind 10
fillet "Fillet5" radius 2 4 edges at (179.65, -140.8544, 1) (190, -140.8544, 1) (50.325, -140.8544, 1) (25, -140.8544, 1)
sketch "Sketch12" plane through (0, 0, 2) normal (0, 0, 1) x (1, 0, 0)
  point P0 (0, 0)
sketch "Sketch13" plane through (0, 0, 2) normal (0, 0, 1) x (1, 0, 0)
  line L0 (22.5889, -109.9594) -> (-89.4111, -109.9594)
  line L1 (-89.4111, -109.9594) -> (-89.4111, -249.9594)
  line L2 (-89.4111, -249.9594) -> (22.5889, -249.9594)
  line L3 (22.5889, -249.9594) -> (22.5889, -109.9594)
  point P0 (0, 0)
  dimension "d160" = 112
  dimension "d161" = 140
  constraints: 8 end point, 2 parallel, 1 horizontal, 1 perpendicular
  measures "d160" distance of L0.start L0.end
  measures "d161" distance of L2.end L0.start
extrude "Extrusion10" add sketch "Sketch13" against normal blind 2
sketch "Sketch14" plane through (0, 0, 2) normal (0, 0, 1) x (1, 0, 0)
  point P0 (0, 0)